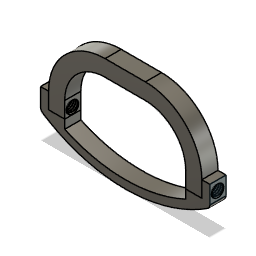
ForeArm v5 (Autodesk Fusion 360 design; units mm, degrees)
Autodesk Fusion 360 part; units mm, degrees
sketch "Sketch1" plane through (0, 0, 0) normal (0, 0, 1) x (1, 0, 0)
  arc A0 (50, 0) -> (25, 25) centre (25, 0) ccw
  line L0 (25, 25) -> (0, 25)
  arc A1 (0, 25) -> (-25, 0) centre (0, 0) ccw
  line L1 (0, 0) -> (25, 0) construction
  arc A2 (60, 0) -> (25, 35) centre (25, 0) ccw
  line L2 (25, 35) -> (0, 35)
  arc A3 (0, 35) -> (-35, 0) centre (0, 0) ccw
  line L3 (-25, 0) -> (-25, -10)
  line L4 (-25, -10) -> (-35, -10)
  line L5 (-35, -10) -> (-35, 0)
  line L6 (60, 0) -> (60, -10)
  line L7 (60, -10) -> (50, -10)
  line L8 (50, -10) -> (50, 0)
  dimension "d1" = 25
  dimension "d2" = 25
  constraint tangent A0 L0
  constraint tangent L0 A1
  constraint horizontal L1
  constraint coincident A1.centre L1.start
  constraint concentric A0 A2
  constraint concentric A1 A3
  constraint tangent A2 L2
  constraint tangent L2 A3
  constraint vertical L3
  constraint horizontal L4
  constraint vertical L5
  constraint vertical L6
  constraint horizontal L7
  constraint vertical L8
  measures "d1" distance of A0.end L0.end
  measures "d2" radius of A1
extrude "Extrude1" add sketch "Sketch1" along normal blind 10 makes body 1
sketch "Sketch2" plane through (0, 0, 10) normal (0, 0, 1) x (1, 0, 0)
  arc A0 (0, 25) -> (-25, 0) centre (0, 0) ccw
  line L0 (0, 25) -> (25, 25)
  arc A1 (50, 0) -> (25, 25) centre (25, 0) ccw
  arc A2 (60, 0) -> (25, 35) centre (25, 0) ccw
  line L1 (25, 35) -> (0, 35)
  arc A3 (0, 35) -> (-35, 0) centre (0, 0) ccw
  line L2 (0, 35) -> (60, 35)
  line L3 (60, 35) -> (60, 25)
  line L4 (60, 25) -> (0, 25)
  line L5 (0, 25) -> (0, 35)
  line L6 (-35, 0) -> (-35, -10)
  line L7 (-35, -10) -> (-25, -10)
  line L8 (-25, -10) -> (-25, 0)
  line L9 (50, 0) -> (50, -10)
  line L10 (50, -10) -> (60, -10)
  line L11 (60, -10) -> (60, 0)
  constraint horizontal L2
  constraint vertical L3
  constraint horizontal L4
  constraint vertical L5
  constraint coincident L1.end A3.start
ref_plane "WorkPlane1" through (85, 0, 0) normal (1, 0, 0) x (0, 1, 0)
sketch "Sketch3" plane through (85, 0, 0) normal (1, 0, 0) x (0, 0, -1)
  circle A0 centre (-5, 0) radius 2.5
  dimension "d12" = 5
  measures "d12" diameter of A0
ref_plane "WorkPlane2" through (30, 0, 0) normal (1, 0, 0) x (0, 1, 0)
sketch "Sketch1 (2)" plane through (0, 0, 10) normal (0, 0, 1) x (1, 0, 0) in component "Component"
  arc A0 (60, 0) -> (25, 35) centre (25, 0) ccw
  line L0 (25, 35) -> (0, 35)
  arc A1 (0, 35) -> (-35, 0) centre (0, 0) ccw
  line L1 (-35, 0) -> (-35, -10)
  line L2 (-35, -10) -> (-25, -10)
  line L3 (-25, -10) -> (-25, 0)
  arc A2 (0, 25) -> (-25, 0) centre (0, 0) ccw
  line L4 (0, 25) -> (25, 25)
  arc A3 (50, 0) -> (25, 25) centre (25, 0) ccw
  line L5 (50, 0) -> (50, -10)
  line L6 (50, -10) -> (60, -10)
  line L7 (60, -10) -> (60, 0)
  line L8 (-40, 0) -> (-35, 0)
  line L9 (-35, 0) -> (-35, -10)
  line L10 (-40, -11.0953) -> (-40, 0)
  line L11 (12.5, 35) -> (12.5, -23.7258)
  line L12 (-63.9415, 43.2021) -> (-45, 30)
  arc A4 (-25, -15.4452) -> (12.5, -23.7258) centre (12.5, 65.3271) ccw
  line L13 (-25, -15.4452) -> (-25, -10)
  line L14 (-35, -10) -> (-25, -10)
  line L15 (12.5, -23.7258) -> (12.5, -28.7258)
  arc A5 (-38.6309, -13.6133) -> (12.5, -28.7258) centre (12.5, 65.3271) ccw
  arc A6 (-40, -11.0953) -> (-38.6309, -13.6133) centre (-37, -11.0953) ccw
  line L16 (65, 0) -> (60, 0)
  line L17 (65, -11.0953) -> (65, 0)
  line L18 (60, 0) -> (60, -10)
  arc A7 (12.5, -28.7258) -> (63.6309, -13.6133) centre (12.5, 65.3271) ccw
  line L19 (60, -10) -> (50, -10)
  line L20 (50, -15.4452) -> (50, -10)
  arc A8 (12.5, -23.7258) -> (50, -15.4452) centre (12.5, 65.3271) ccw
  arc A9 (63.6309, -13.6133) -> (65, -11.0953) centre (62, -11.0953) ccw
  dimension "d23" = 5
  dimension "d26" = 3
  dimension "d27" = 3
  constraint horizontal L8
  constraint vertical L9
  constraint vertical L10
  constraint coincident L1.end L2.start
  constraint midpoint L0 L11.start
  constraint perpendicular L0 L11
  constraint coincident L2.end L3.start
  constraint parallel L11 L15
  constraint concentric A4 A5
  constraint tangent A5 A6
  constraint tangent L10 A6
  constraint vertical L13
  constraint symmetric L8.start L11 L16.start
  constraint symmetric A1.end L11 A0.start
  constraint symmetric L1.end L11 L6.end
  constraint symmetric A4.end L11 L15.start
  constraint symmetric L11 A4 A8
  constraint symmetric L11 A4.start L20.start
  constraint symmetric L11 L2.end L5.end
  constraint symmetric L11 L15.end A5.end
  constraint symmetric L11 A5 A7
  constraint tangent A7 A9
  constraint tangent L17 A9
  measures "d23" distance of L8.start A1.end
  measures "d26" radius of A6
  measures "d27" radius of A9
extrude "Extrude1'" add sketch "Sketch1 (2)" against normal blind 10 separate body contours L6 L7 L15 L16 L17 L18 A7 L19 L20 A8 A9 | L1 L2 L8 L9 L10 A4 L13 L14 L15 A5 A6 makes body 2 in component "Component"
sketch "Sketch5" plane through (65, 0, 0) normal (1, 0, 0) x (0, 0, -1)
  line L0 (-10, 0) -> (-10, -11.0953)
  line L1 (-10, -11.0953) -> (0, -11.0953)
  line L2 (0, -11.0953) -> (0, 0)
  line L3 (0, 0) -> (-10, 0)
sketch "Sketch2 (2)" plane through (65, -5.5477, 5) normal (1, 0, 0) x (0, 0, -1) in component "Component"
  circle A0 centre (0, 0) radius 4
  dimension "d30" = 8
  constraint coincident A0.centre origin
  measures "d30" diameter of A0
extrude "Extrude7" cut sketch "Sketch2 (2)" against normal blind 136 bodies 1
extrude "Extrude2" cut sketch "Sketch2 (2)" against normal blind 136 bodies 2 in component "Component"
thread "Thread1" "ISO Metric profile 8.0 M8x1.25 6H" major diameter 8.17 minor diameter 6.7795 pitch 1.25 angle 60 modelled right hand crest width 0.343 on face at (-36.6667, -5.9459, 1.0199) crest through (-35.3125, -5.5477, 1.6102) on bodies 2 in component "Component"
thread "Thread3" "ISO Metric profile 8.0 M8x1.25 6H" major diameter 8.17 minor diameter 6.7795 pitch 1.25 angle 60 modelled right hand crest width 0.343 on face at (-28.3333, -5.9459, 1.0199) crest through (-25.3125, -5.5477, 1.6102) on bodies 1
thread "Thread2" "ISO Metric profile 8.0 M8x1.25 6H" major diameter 8.17 minor diameter 6.7795 pitch 1.25 angle 60 modelled right hand crest width 0.343 on face at (63.3333, -5.9459, 1.0199) crest through (64.6875, -5.5477, 1.6102) on bodies 2 in component "Component"
thread "Thread4" "ISO Metric profile 8.0 M8x1.25 6H" major diameter 8.17 minor diameter 6.7795 pitch 1.25 angle 60 modelled right hand crest width 0.343 on face at (56.6667, -5.9459, 1.0199) crest through (59.6875, -5.5477, 1.6102) on bodies 1
component "Component" placed x (1, 0, 0) y (0, 1, 0) z (0, 0, 1) at (0, 0, 0)
equation "d1 = 60 mm - 35 mm"
